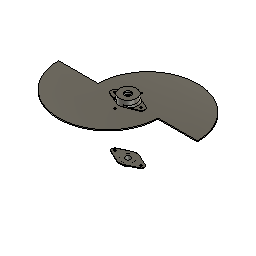
Savonius Turbine (Autodesk Fusion 360 design; units mm, degrees)
Autodesk Fusion 360 part; units mm, degrees
note: some values were not read from the file. Chosen so that the rebuilt part matches the saved one: a direction; which face or edge a step refers to; which pieces of a blend or face edit are solid. Set by a fixed rule: which sketch regions a step uses.
sketch "Sketch1" plane through (0, 0, 0) normal (0, 0, 1) x (1, 0, 0) in component "Turbine"
  line L0 (105, 0) -> (-105, 0)
  arc A0 (-105, 0) -> (45, 0) centre (-30, 0) ccw
  arc A1 (105, 0) -> (-45, 0) centre (30, 0) ccw
  arc A2 (104.6, 0) -> (-44.6, 0) centre (30, 0) ccw
  arc A3 (-104.6, 0) -> (44.6, 0) centre (-30, 0) ccw
  line L1 (0, 0) -> (0, -20) construction
  circle A4 centre (0, 0) radius 11.5
  circle A5 centre (0, -20) radius 1.5
  circle A6 centre (20, 0) radius 1.5
  circle A7 centre (0, 20) radius 1.5
  circle A8 centre (-20, 0) radius 1.5
  dimension "d4" = 150
  dimension "d5" = 60
  dimension "d6" = -0.4
  dimension "d7" = -0.4
  dimension "d17" = 23
  dimension "d31" = 20
  dimension "d44" = 360
  constraint horizontal L0
  constraint midpoint L1.start L0
  constraint coincident L0 A0.centre
  constraint coincident L0 A1.centre
  constraint equal A0 A1
  constraint coincident L0 A0.end
  constraint coincident L0 A1.end
  constraint coincident L1.start A4.centre
  constraint perpendicular L0 L1
  constraint coincident L1.end A5.centre
  measures "d4" diameter of A0
  measures "d5" distance of A0.centre A1.centre
  measures "d17" diameter of A4
  measures "d31" distance of L1.start L1.end
extrude "Extrude1" add sketch "Sketch1" along normal blind 1.6 contours L0 A2 A4 A6 A8 | L0 A3 A4 A6 A8 makes body 1 in component "Turbine"
extrude "Extrude2" add sketch "Sketch1" along normal blind 75 contours L0 A1 A2 | L0 A0 A3 bodies 1 in component "Turbine"
extrude "Extrude3" add sketch "Sketch1" against normal blind 1.6 from surface at 75 separate body contours L0 A1 A2 | L0 A2 A4 A6 A8 | L0 A3 A4 A6 A8 | L0 A0 A3 makes body 2 in component "Turbine"
sketch "Sketch1 (2)" plane through (0, 0, 75) normal (0, 0, 1) x (-1, 0, 0) in component "Bearing Cap"
  circle A0 centre (0, 0) radius 11.5
  line L0 (-45, 0) -> (-105, 0)
  arc A1 (-105, 0) -> (45, 0) centre (-30, 0) ccw
  line L1 (45, 0) -> (105, 0)
  arc A2 (105, 0) -> (-45, 0) centre (30, 0) ccw
  circle A3 centre (0, 0) radius 11.5
  line L2 (-105, 0) -> (105, 0)
  circle A4 centre (0, 0) radius 11
  circle A5 centre (0, 0) radius 5
  circle A6 centre (0, 0) radius 13
  circle A7 centre (-20, 0) radius 5.5
  line L3 (22.0625, -5.0986) -> (4.875, -12.0513)
  line L4 (-4.875, -12.0513) -> (-22.0625, -5.0986)
  line L5 (22.0625, 5.0986) -> (4.875, 12.0513)
  line L6 (-4.875, 12.0513) -> (-22.0625, 5.0986)
  circle A8 centre (0, 20) radius 1.5
  circle A9 centre (-20, 0) radius 1.5
  circle A10 centre (0, -20) radius 1.5
  circle A11 centre (20, 0) radius 5.5
  circle A12 centre (20, 0) radius 1.5
  circle A13 centre (0, -20) radius 1.5
  circle A14 centre (20, 0) radius 1.5
  circle A15 centre (-20, 0) radius 1.5
  point P0 (20, 0)
  dimension "d19" = 10
  dimension "d20" = 22
  dimension "d21" = 2
  dimension "d45" = 4
  constraint coincident A0.centre A3.centre
  constraint concentric A3 A5
  constraint coincident A6 L3.end
  constraint tangent A6 L3
  constraint coincident A6 L4.start
  constraint coincident A7 L4.end
  constraint tangent A7 L4
  constraint symmetric L2 L3.start L5.start
  constraint symmetric L2 L3.end L5.end
  constraint symmetric L2 L4.start L6.start
  constraint symmetric L2 L4.end L6.end
  constraint tangent A6 L4
  constraint coincident P0 A11.centre
  constraint coincident L5.start A11
  constraint tangent L5 A11
  constraint equal A7 A11
  measures "d19" diameter of A5
  measures "d20" diameter of A4
  measures "d45" distance of A7 A9
extrude "Extrude1'" add sketch "Sketch1 (2)" along normal blind 1 separate body contours L2 A6 L5 A11 | L2 A6 L3 A11 | L2 A6 A7 L4 | L2 A6 A7 L6 | L2 A11 A12 A14 | L2 A11 A12 A14 | L2 A7 A9 A15 | L2 A7 A9 A15 makes body 3 at (-17.915, -3.3991, 75) makes body 4 at (17.915, -3.3991, 75) in component "Bearing Cap"
extrude "Extrude2'" add sketch "Sketch1 (2)" along normal blind 7.2 contours A0 A3 L2 A4 | A0 A3 L2 A6 | A0 A3 L2 A4 | A0 A3 L2 A6 bodies 3 4 in component "Bearing Cap"
sketch "Sketch2" plane through (0, 0, 82.2) normal (0, 0, 1) x (-1, 0, 0) in component "Bearing Cap"
  circle A0 centre (0, 0) radius 11
  circle A1 centre (0, 0) radius 13
  circle A2 centre (0, 0) radius 13
  circle A3 centre (0, 0) radius 5
extrude "Extrude5" add sketch "Sketch2" along normal blind 2.3 contours A0 | A1 A2 bodies 3 in component "Bearing Cap"
sketch "Sketch1 (3)" plane through (0, 0, 75) normal (0, 0, 1) x (-1, 0, 0) in component "Solid 8mm shaft mount"
  circle A0 centre (0, 0) radius 11.5
  line L0 (-45, 0) -> (-105, 0)
  arc A1 (-105, 0) -> (45, 0) centre (-30, 0) ccw
  line L1 (45, 0) -> (105, 0)
  arc A2 (105, 0) -> (-45, 0) centre (30, 0) ccw
  circle A3 centre (0, 0) radius 11.5 construction
  circle A4 centre (20, 0) radius 1.5
  circle A5 centre (-20, 0) radius 1.5
  line L2 (-105, 0) -> (105, 0) construction
  circle A6 centre (0, 0) radius 11 construction
  circle A7 centre (0, 0) radius 4
  circle A8 centre (0, 0) radius 13
  circle A9 centre (-20, 0) radius 4.5
  line L3 (21.9125, -4.0734) -> (5.525, -11.7675)
  line L4 (-5.525, -11.7675) -> (-21.9125, -4.0734)
  line L5 (21.9125, 4.0734) -> (5.525, 11.7675)
  line L6 (-5.525, 11.7675) -> (-21.9125, 4.0734)
  circle A10 centre (0, 20) radius 1.5
  circle A11 centre (0, 0) radius 8
  circle A12 centre (20, 0) radius 4.5
  circle A13 centre (0, -20) radius 1.5
  circle A14 centre (20, 0) radius 1.5
  circle A15 centre (-20, 0) radius 1.5
  dimension "d19_1" = 8
  dimension "d20_1" = 22
  dimension "d21_1" = 2
  dimension "d22_1" = 3
  dimension "d36" = 4
  constraint coincident A0.centre A3.centre
  constraint concentric A3 A7
  constraint coincident A8 L3.end
  constraint tangent A8 L3
  constraint coincident A8 L4.start
  constraint coincident A9 L4.end
  constraint tangent A9 L4
  constraint symmetric L2 L3.start L5.start
  constraint symmetric L2 L3.end L5.end
  constraint symmetric L2 L4.start L6.start
  constraint symmetric L2 L4.end L6.end
  constraint tangent A8 L4
  constraint concentric A3 A11
  constraint concentric A4 A12
  constraint coincident L5.start A12
  measures "d19_1" diameter of A7
  measures "d20_1" diameter of A6
  measures "d22_1" distance of A5
  measures "d36" distance of A7 A11
extrude "Extrude1''" add sketch "Sketch1 (3)" along normal blind 1 separate body contours A0 | A8 | A8 L3 L5 A12 | A8 A9 L4 L6 | A12 | A9 makes body 5 in component "Solid 8mm shaft mount"
extrude "Extrude4" add sketch "Sketch1 (3)" along normal blind 6 contours A11 bodies 5 in component "Solid 8mm shaft mount"
ref_plane "WorkPlane1" through (0, 8, 79.0362) normal (0, 1, 0) x (1, 0, 0) in component "Solid 8mm shaft mount"
sketch "Sketch2 (2)" plane through (0, 8, 0) normal (0, 1, 0) x (1, 0, 0) in component "Solid 8mm shaft mount"
  line L0 (-8, -81) -> (8, -81)
  line L1 (-5.525, -75) -> (5.525, -75)
  line L2 (-5.525, -75) -> (-5.525, -76)
  line L3 (-5.525, -76) -> (5.525, -76)
  line L4 (5.525, -76) -> (5.525, -75)
  line L5 (0, -81) -> (0, -76) construction
  circle A0 centre (0, -78.5) radius 1.4
  dimension "d40" = 2.8
  constraint midpoint L0 L5.start
  constraint midpoint L3 L5.end
  constraint midpoint L5 A0.centre
  measures "d40" diameter of A0
extrude "Extrude5'" cut sketch "Sketch2 (2)" against normal blind 8 contours A0 bodies 5 in component "Solid 8mm shaft mount"
chamfer "Chamfer1" distance 2 angle 45 3 edges at (-10.779, 7.2672, 76) (13, 0, 76) (-10.779, -7.2672, 76) on bodies 3 in component "Bearing Cap"
sketch "Sketch3" plane through (0, 0, 82.2) normal (0, 0, -1) x (1, 0, 0) in component "Bearing Cap"
  circle A0 centre (0, 0) radius 5
  circle A1 centre (0, 0) radius 11
  line L0 (-9.798, -5) -> (9.798, -5)
  line L1 (0, 0) -> (-2.9724, 0) construction
  line L2 (-9.798, 5) -> (9.798, 5)
  line L3 (5, -5) -> (5, 5)
  line L4 (-5, -5) -> (-5, 5)
  constraint coincident A1 L0.start
  constraint coincident A1 L0.end
  constraint horizontal L0
  constraint coincident A0.centre A1.centre
  constraint horizontal L1
  constraint symmetric L0.start L1 L2.start
  constraint symmetric L0.end L1 L2.end
  constraint tangent A0 L0
  constraint coincident L0 L3.start
  constraint coincident L2 L3.end
  constraint perpendicular L2 L3
  constraint coincident L0 L4.start
  constraint coincident L2 L4.end
  constraint perpendicular L2 L4
  constraint tangent A0 L3
  constraint tangent A0 L4
extrude "Extrude6" cut sketch "Sketch3" against normal blind 0.4 contours A0 L0 L3 | A1 L0 L2 L3 | A0 L2 L3 | A0 L2 L4 | A0 L0 L4 | A1 L0 L2 L4 bodies 3 in component "Bearing Cap"
extrude "Extrude7" cut sketch "Sketch3" against normal blind 0.6 contours A0 L0 L3 | A0 L2 L3 | A0 L2 L4 | A0 L0 L4 bodies 3 in component "Bearing Cap"
chamfer "Chamfer1'" distance 1 angle 45 1 edges at (7.4586, -2.8929, 76) on bodies 5 in component "Solid 8mm shaft mount"
component "Turbine" placed x (1, 0, 0) y (0, 1, 0) z (0, 0, 1) at (0, 0, 0)
component "Bearing Cap" placed x (1, 0, 0) y (0, 1, 0) z (0, 0, 1) at (0, 0, 0) in component "Turbine"
component "Solid 8mm shaft mount" placed x (1, 0, 0) y (0, -1, 0) z (0, 0, -1) at (0, 0, 75) in component "Turbine"
hidden bodies 1
equation "d5 = d4 * 0.4"
named bodies: "Turbine body main", "Turbine body cap", "608Bearing mount", "Solid 8mm shaft mount"
